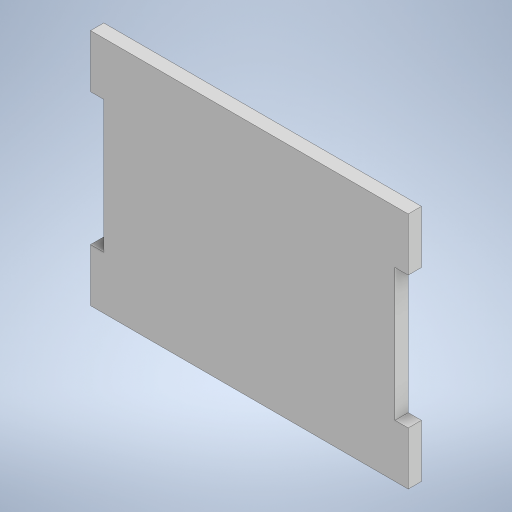
# Autodesk Inventor part: bottomside
Saved by Autodesk Inventor 2024 (Build 280153000, 153)
## iProperties
Created: 2024-04-16
Part Number: bottomside
Material: Generic
Document SubType Name: Modeling
Designer: srika
Density: 1 g/cm^3
Appearance: Default
Author: srika
Autodesk Inventor part; units mm, degrees
ref_plane "YZ Plane" through (0, 0, 0) normal (1, 0, 0) x (0, 1, 0)
ref_plane "XZ Plane" through (0, 0, 0) normal (0, 1, 0) x (-1, 0, 0)
ref_plane "XY Plane" through (0, 0, 0) normal (0, 0, 1) x (1, 0, 0)
sketch "Sketch1" plane through (0, 0, 0) normal (0, 0, 1) x (1, 0, 0)
  line L0 (5, 5) -> (115, 5)
  line L1 (115, 5) -> (115, 95)
  line L2 (115, 95) -> (5, 95)
  line L3 (5, 95) -> (5, 5)
  line L4 (0, 25) -> (5, 25)
  line L5 (5, 25) -> (5, 5)
  line L6 (5, 5) -> (0, 5)
  line L7 (0, 5) -> (0, 25)
  line L8 (0, 95) -> (5, 95)
  line L9 (5, 95) -> (5, 75)
  line L10 (5, 75) -> (0, 75)
  line L11 (0, 75) -> (0, 95)
  line L12 (120, 95) -> (115, 95)
  line L13 (115, 95) -> (115, 75)
  line L14 (115, 75) -> (120, 75)
  line L15 (120, 75) -> (120, 95)
  line L16 (120, 5) -> (115, 5)
  line L17 (115, 5) -> (115, 25)
  line L18 (115, 25) -> (120, 25)
  line L19 (120, 25) -> (120, 5)
  constraints: 40 end point, 10 parallel, 10 point on line, 5 horizontal, 5 perpendicular
extrude "Extrusion2" add sketch "Sketch1" along normal blind 5
body "Solid2"
